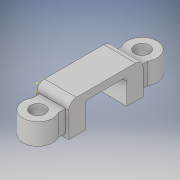
# Autodesk Inventor part: HP45 Printhead Cap
Saved by Autodesk Inventor 2018 (Build 220112000, 112)
## iProperties
Created: 2018-03-13
Part Number: HP45 Printhead Cap
Material: Generic
Document SubType Name: Modeling
Designer: junai
Density: 1 g/cm^3
Appearance: Default
Author: junai
Autodesk Inventor part; units mm, degrees
note: some values were not read from the file. Chosen so that the rebuilt part matches the saved one: sketch regions of "Extrusion4".
ref_plane "YZ Plane" through (0, 0, 0) normal (1, 0, 0) x (0, 1, 0)
ref_plane "XZ Plane" through (0, 0, 0) normal (0, 1, 0) x (-1, 0, 0)
ref_plane "XY Plane" through (0, 0, 0) normal (0, 0, 1) x (1, 0, 0)
sketch "Sketch1" plane through (0, 0, 0) normal (1, 0, 0) x (0, 1, 0)
  point P0 (0, 0)
sketch "Sketch2" plane through (0, 0, 0) normal (0, 1, 0) x (-1, 0, 0)
  point P0 (0, 0)
sketch "Sketch3" plane through (0, 0, 0) normal (0, 1, 0) x (-1, 0, 0)
  line L0 (0, 0) -> (-15, 0)
  line L1 (-15, 0) -> (-15, -35)
  line L2 (-15, -35) -> (0, -35)
  line L3 (0, -35) -> (0, 0)
  dimension "d0" = 35
  dimension "d1" = 15
  constraints: 8 end point, 2 parallel, 1 horizontal, 1 perpendicular
  measures "d0" distance of L0.end L1.end
  measures "d1" distance of L1.end L2.end
extrude "Extrusion1" add sketch "Sketch3" along normal blind 3.5
sketch "Sketch4" plane through (0, 0, 0) normal (0, -1, 0) x (1, 0, 0)
  point P0 (0, 0)
sketch "Sketch5" plane through (0, 0, 0) normal (0, -1, 0) x (1, 0, 0)
  line L0 (15, 0) -> (15, -35) projected
  line L1 (15, 0) -> (0, 0)
  line L2 (0, 0) -> (0, -6.5)
  line L3 (0, -6.5) -> (15, -6.5)
  line L4 (15, -6.5) -> (15, 0)
  line L5 (0, -35) -> (0, 0) projected
  line L6 (15, -35) -> (0, -35)
  line L7 (0, -35) -> (0, -28.5)
  line L8 (0, -28.5) -> (15, -28.5)
  line L9 (15, -28.5) -> (15, -35)
  dimension "d4" = 6.5
  dimension "d5" = 6.5
  constraints: 16 end point, 4 parallel, 2 horizontal, 2 perpendicular, 1 collinear, 1 point on line
  measures "d4" distance of L1.end L2.end
  measures "d5" distance between parallel lines of L6 L8
extrude "Extrusion2" add sketch "Sketch5" along normal blind 12 contours L0 L3 L2 L1 | L0 L6 L5 L8
fillet "Fillet2" radius 3.5875 2 edges at (7.5, 3.5, -35) (7.5, 3.5, 0)
sketch "Sketch7" plane through (0, 3.5, 0) normal (0, 1, 0) x (1, 0, 0)
  point P0 (0, 0)
sketch "Sketch8" plane through (0, -12, 0) normal (0, -1, 0) x (1, 0, 0)
  circle A0 centre (7.5, 7) radius 7
  circle A1 centre (7.5, -42) radius 7
  line L0 (15, 0) -> (0, 0) projected
  line L1 (0, -35) -> (15, -35) projected
  circle A2 centre (7.5, 7) radius 3.5
  circle A3 centre (7.5, -42) radius 3.5
  line L2 (0, 0) -> (15, 0) projected
  line L3 (13.5622, 0) -> (1.4378, 0)
  line L4 (1.4378, 0) -> (1.4378, 3.5)
  line L5 (1.4378, 3.5) -> (13.5622, 3.5)
  line L6 (13.5622, 3.5) -> (13.5622, 0)
  line L7 (13.5622, -35) -> (1.4378, -35)
  line L8 (1.4378, -35) -> (1.4378, -38.5)
  line L9 (1.4378, -38.5) -> (13.5622, -38.5)
  line L10 (13.5622, -38.5) -> (13.5622, -35)
  point P0 (7.5, 0)
  point P1 (7.5, -35)
  dimension "d14" = 14
  dimension "d15" = 14
  dimension "d16" = 7
  dimension "d17" = 7
  constraints: 16 end point, 6 point on circle, 4 centre point, 4 parallel, 4 tangent, 2 coincident, 2 horizontal, 2 midpoint, 2 perpendicular, 2 point on line
  measures "d14" diameter of A0
  measures "d15" diameter of A1
  measures "d16" diameter of A2
  measures "d17" diameter of A3
extrude "Extrusion4" add sketch "Sketch8" against normal blind 12 contours A0 L5 | L5 A0 | L6 L0 A0 | A1 L9 | L9 A1 | A1 L1 L10 | L8 L1 A1
sketch "Sketch9" plane through (0, -12, 0) normal (0, -1, 0) x (1, 0, 0)
  line L0 (7.5, 0) -> (13.5622, 0) projected
  line L1 (7.5, 0) -> (1.4378, 0)
  line L2 (1.4378, 0) -> (1.4378, 3.5)
  line L3 (1.4378, 3.5) -> (7.5, 3.5)
  line L4 (7.5, 3.5) -> (7.5, 0)
  arc A0 (13.5622, 3.5) -> (7.5, 0) centre (7.5, 7) ccw projected
  point P0 (0, 0)
  constraints: 8 end point, 2 parallel, 1 horizontal, 1 perpendicular, 1 point on circle
extrude "Extrusion5" add sketch "Sketch9" against normal blind 12
sketch "Sketch10" plane through (0, -12, 0) normal (0, -1, 0) x (1, 0, 0)
  line L0 (15, 0) -> (13.5622, 0) projected
  line L1 (15, 0) -> (0, 0)
  line L2 (0, 0) -> (0, 14.6227)
  line L3 (0, 14.6227) -> (15, 14.6227)
  line L4 (15, 14.6227) -> (15, 0)
  line L5 (15, -31.4125) -> (15, -35) projected
  line L6 (15, -35) -> (0, -35)
  line L7 (0, -35) -> (0, -49.9262)
  line L8 (0, -49.9262) -> (15, -49.9262)
  line L9 (15, -49.9262) -> (15, -35)
  point P0 (0, 0)
  constraints: 16 end point, 4 parallel, 2 horizontal, 2 perpendicular, 1 point on line
extrude "Extrusion6" cut sketch "Sketch10" against normal blind 2
sketch "Sketch11" plane through (0, -12, 0) normal (0, -1, 0) x (1, 0, 0)
  line L0 (0, -6.5) -> (15, -6.5) projected
  line L1 (0, -6.5) -> (15, -6.5)
  line L2 (15, -6.5) -> (15, -7.7)
  line L3 (15, -7.7) -> (0, -7.7)
  line L4 (0, -7.7) -> (0, -6.5)
  line L5 (15, -6.5) -> (15, -28.5) projected
  line L6 (0, -28.5) -> (0, -6.5) projected
  line L7 (15, -28.5) -> (0, -28.5)
  line L8 (0, -28.5) -> (0, -27.3)
  line L9 (0, -27.3) -> (15, -27.3)
  line L10 (15, -27.3) -> (15, -28.5)
  point P0 (0, 0)
  dimension "d24" = 1.2
  dimension "d25" = 1.2
  constraints: 16 end point, 4 parallel, 2 horizontal, 2 perpendicular, 1 point on line
  measures "d24" distance of L1.end L2.end
  measures "d25" distance between parallel lines of L7 L9
extrude "Extrusion7" add sketch "Sketch11" against normal blind 12 contours L0 L2 L3 L4 | L9 L5 L7 L6
fillet "Fillet4" radius 2 2 edges at (7.5, 0, -7.7) (7.5, 0, -27.3)
body "Solid1"
